Autodesk Fusion 360 part; units mm, degrees
note: some values were not read from the file. Chosen so that the rebuilt part matches the saved one: which pieces of a blend or face edit are solid.
(part 2 of 5)
  measures "d848" distance of L239.end L236.start
  measures "d854" distance of L244.start L244.end
  measures "d856" distance of L244.start L246.start
  measures "d862" distance of L237.end L256.start
  measures "d867" distance of L243.end L255.start
  measures "d868" distance of L255 L256
  measures "d884" distance of L393.end L393.start
  measures "d885" distance of L393.start L392.end
  measures "d887" distance of L392.start L392.end
  measures "d890" distance of L400.end L412.end
  measures "d896" distance of L150 L164
  measures "d921" distance of L177.start P8
  measures "d922" distance of L177 L458
  measures "d923" distance of L453 L458
  measures "d929" distance of L171.start L469.start
  measures "d930" distance of L171.start L23.end
  measures "d931" distance of P6 L472.start
  measures "d932" distance of P6 L473.end
  measures "d933" distance of L23 L24
  measures "d934" distance of L55.start L476.end
  measures "d937" distance of L7.start L57.end
  measures "d938" distance of L169 L479
  measures "d948" distance of L49.end L481.end
  measures "d949" distance of L482.start L482.end
  measures "d951" distance of L4.start L502.start
  measures "d956" distance of L172 L179
  measures "d1024" diameter of A16
  measures "d1025" diameter of A17
  measures "d1031" distance of L523 L524
sketch "Skizze2" plane through (0, 0, 0) normal (0, 0, 1) x (1, 0, 0)
  line L0 (0, 7.8901) -> (0, 0)
  line L1 (250, 0) -> (250, 8)
  line L2 (10, 8) -> (10, 0)
  line L3 (0, 0) -> (10, 0)
  line L4 (34.8226, 77.9951) -> (0.2007, 77.9951)
  line L5 (4.5, -4.5) -> (245.5, -4.5)
  line L6 (245.5, -245.5) -> (4.5, -245.5)
  line L7 (4.5, -245.5) -> (4.5, -4.5)
  circle A0 centre (7.5, -7.5) radius 1.5
  circle A1 centre (7.5, -7.5) radius 1.5
  circle A2 centre (7.7007, 70.4951) radius 1.5
  line L8 (240, 8) -> (10, 8)
  line L9 (240, 8) -> (240, 0)
  line L10 (0, 0) -> (0, 7.8901)
  line L11 (34.8226, 85.9951) -> (34.8226, 77.9951)
  line L12 (188.7268, 54.5014) -> (175.7207, 54.4951)
  line L13 (175.7207, 54.4951) -> (175.7307, 61.495)
  line L14 (175.7307, 61.495) -> (188.7307, 61.4887)
  line L15 (188.7307, 61.4887) -> (188.7268, 54.5014)
  line L16 (170.2913, 54.4924) -> (157.2903, 54.4861)
  line L17 (157.2903, 54.4861) -> (157.3035, 61.4861)
  line L18 (157.3035, 61.4861) -> (170.3035, 61.4612)
  line L19 (170.3035, 61.4612) -> (170.2913, 54.4924)
  line L20 (150.7313, 54.5045) -> (135.7242, 54.4951)
  line L21 (135.7242, 54.4951) -> (135.7359, 61.495)
  line L22 (135.7359, 61.495) -> (150.7359, 61.4856)
  line L23 (150.7359, 61.4856) -> (150.7313, 54.5045)
  line L24 (121.7084, 53.9672) -> (108.2084, 53.9709)
  line L25 (108.2084, 53.9709) -> (106.7182, 62.0188)
  line L26 (106.7182, 62.0188) -> (123.2182, 62.0233)
  line L27 (123.2182, 62.0233) -> (121.7084, 53.9672)
  line L28 (31.2246, 51.4951) -> (19.7246, 51.5056)
  line L29 (19.7246, 51.5056) -> (19.7282, 64.4845)
  line L30 (19.7282, 64.4845) -> (31.2439, 64.4951)
  line L31 (31.2439, 64.4951) -> (31.2246, 51.4951)
  circle A3 centre (18.2368, 25.8861) radius 4
  line L32 (211.2035, 57.9951) -> (16.1921, 57.9951)
  line L33 (95.7998, 57.9951) -> (36.1928, 58.2134)
  line L34 (36.1928, 58.2134) -> (36.1928, 40.7134)
  line L35 (36.1928, 40.7134) -> (95.799, 40.4951)
  line L36 (95.799, 40.4951) -> (95.7998, 57.9951)
  line L37 (47.3226, 85.9941) -> (47.3226, 77.9951)
  line L38 (90.3666, 86) -> (90.3677, 77.9951)
  line L39 (102.8855, 86) -> (102.8844, 77.9951)
  line L40 (145.9318, 86) -> (145.9321, 77.9951)
  line L41 (158.4356, 86) -> (158.4355, 77.9951)
  line L42 (201.4887, 86) -> (201.4887, 77.9951)
  line L43 (213.9898, 86) -> (213.9897, 77.9951)
  line L44 (47.3226, 85.9941) -> (34.8226, 85.9951)
  line L45 (102.8855, 86) -> (90.3666, 86)
  line L46 (158.4356, 86) -> (145.9318, 86)
  line L47 (213.9898, 86) -> (201.4887, 86)
  line L48 (-7.8996, 42.9426) -> (-7.8996, 7.8901)
  line L49 (-7.8996, 7.8901) -> (0, 7.8901)
  line L50 (250.1004, 77.9951) -> (258.1004, 77.9951)
  line L51 (258.1004, 8) -> (250, 8)
  circle A4 centre (242.7007, 70.4951) radius 1.5
  circle A5 centre (7.7007, 15.4951) radius 1.5
  circle A6 centre (242.7007, 15.4951) radius 1.5
  line L52 (213.9897, 77.9951) -> (250.1004, 77.9951)
  line L53 (213.9897, 77.9951) -> (250.1004, 77.9951)
  line L54 (158.4355, 77.9951) -> (201.4887, 77.9951)
  line L55 (158.4355, 77.9951) -> (201.4887, 77.9951)
  line L56 (102.8844, 77.9951) -> (145.9321, 77.9951)
  line L57 (47.3226, 77.9951) -> (90.3677, 77.9951)
  line L58 (102.8844, 77.9951) -> (145.9321, 77.9951)
  line L59 (0.2007, 77.9951) -> (34.8226, 77.9951)
  line L60 (47.3226, 77.9951) -> (90.3677, 77.9951)
  line L61 (0.1004, 369.8881) -> (-7.8996, 369.8881)
  line L62 (240.1004, 379.8881) -> (240.1004, 387.8881)
  line L63 (222.2222, 129.8881) -> (222.2222, 121.8881)
  line L64 (27.7778, 129.8881) -> (27.7778, 121.8881)
  line L65 (111.1111, 129.8881) -> (111.1111, 121.8881)
  line L66 (138.8889, 129.8881) -> (138.8889, 121.8881)
  line L67 (55.5556, 129.8881) -> (55.5556, 121.8881)
  line L68 (194.4444, 129.8881) -> (194.4444, 121.8881)
  circle A7 centre (7.6004, 137.3881) radius 1.5
  line L69 (166.6667, 129.8881) -> (166.6667, 121.8881)
  line L70 (0, 129.8881) -> (0, 121.8881)
  line L71 (83.3333, 129.8881) -> (83.3333, 121.8881)
  line L72 (-7.8996, 369.8881) -> (-7.8996, 139.8881)
  circle A8 centre (242.6004, 137.3881) radius 1.5
  line L73 (10.1004, 387.8881) -> (10.1004, 379.8881)
  circle A9 centre (242.6004, 372.3881) radius 1.5
  line L74 (240.1004, 387.8881) -> (10.1004, 387.8881)
  line L75 (0, 139.8881) -> (0, 129.8881)
  line L76 (-7.8996, 139.8881) -> (0, 139.8881)
  line L77 (240.1004, 379.8881) -> (250.1004, 379.8881)
  line L78 (0.1004, 379.8881) -> (10.1004, 379.8881)
  line L79 (0.1004, 379.8881) -> (0.1004, 369.8881)
  circle A10 centre (7.6004, 372.3881) radius 1.5
  line L80 (240, 0) -> (250, 0)
  line L81 (10, 0) -> (0, 0)
  circle A11 centre (7.5, -14.4118) radius 1.5
  circle A12 centre (7.5, -21.3235) radius 1.5
  circle A13 centre (7.5, -28.2353) radius 1.5
  circle A14 centre (7.5, -35.1471) radius 1.5
  circle A15 centre (7.5, -42.0588) radius 1.5
  circle A16 centre (7.5, -48.9706) radius 1.5
  circle A17 centre (7.5, -55.8824) radius 1.5
  circle A18 centre (7.5, -62.7941) radius 1.5
  circle A19 centre (7.5, -69.7059) radius 1.5
  circle A20 centre (7.5, -76.6176) radius 1.5
  circle A21 centre (7.5, -83.5294) radius 1.5
  circle A22 centre (7.5, -90.4412) radius 1.5
  circle A23 centre (7.5, -97.3529) radius 1.5
  circle A24 centre (7.5, -104.2647) radius 1.5
  circle A25 centre (7.5, -111.1765) radius 1.5
  circle A26 centre (7.5, -118.0882) radius 1.5
  circle A27 centre (7.5, -125) radius 1.5
  circle A28 centre (7.5, -131.9118) radius 1.5
  circle A29 centre (7.5, -138.8235) radius 1.5
  circle A30 centre (7.5, -145.7353) radius 1.5
  circle A31 centre (7.5, -152.6471) radius 1.5
  circle A32 centre (7.5, -159.5588) radius 1.5
  circle A33 centre (7.5, -166.4706) radius 1.5
  circle A34 centre (7.5, -173.3824) radius 1.5
  circle A35 centre (7.5, -180.2941) radius 1.5
  circle A36 centre (7.5, -187.2059) radius 1.5
  circle A37 centre (7.5, -194.1176) radius 1.5
  circle A38 centre (7.5, -201.0294) radius 1.5
  circle A39 centre (7.5, -207.9412) radius 1.5
  circle A40 centre (7.5, -214.8529) radius 1.5
  circle A41 centre (7.5, -221.7647) radius 1.5
  circle A42 centre (7.5, -228.6765) radius 1.5
  circle A43 centre (7.5, -235.5882) radius 1.5
  circle A44 centre (7.5, -242.5) radius 1.5
  circle A45 centre (170.8722, -303.1832) radius 1.75
  circle A46 centre (170.8722, -273.1832) radius 1.75
  circle A47 centre (95.8722, -273.1832) radius 1.75
  line L82 (245.5, -323.5) -> (4.5, -323.5)
  circle A48 centre (60.4769, -288.1832) radius 8
  line L83 (245.5, -262.5) -> (245.5, -323.5)
  circle A49 centre (79.6349, -288.1832) radius 3.25
  line L84 (97.6222, -276.9332) -> (169.1222, -276.9332)
  line L85 (169.1222, -299.4332) -> (97.6222, -299.4332)
  line L86 (169.1222, -276.9332) -> (169.1222, -299.4332)
  circle A50 centre (95.8722, -303.1832) radius 1.75
  line L87 (97.6222, -299.4332) -> (97.6222, -276.9332)
  line L88 (4.5, -323.5) -> (4.5, -262.5)
  line L89 (4.5, -262.5) -> (245.5, -262.5)
  circle A51 centre (7.5, -265.5) radius 1.5
  circle A52 centre (7.5, -265.5) radius 1.5
  circle A53 centre (19.25, -265.5) radius 1.5
  circle A54 centre (7.5, -274.6667) radius 1.5
  circle A55 centre (19.25, -274.6667) radius 1.5
  line L90 (-12.5, -4.5) -> (-73.5, -4.5)
  line L91 (-12.5, -245.5) -> (-12.5, -4.5)
  circle A56 centre (235, -284.5) radius 3
  circle A57 centre (235, -272.5) radius 3
  line L92 (229, -215.5) -> (231, -215.5)
  line L93 (231, -215.5) -> (231, -239.5)
  line L94 (231, -239.5) -> (229, -239.5)
  line L95 (229, -239.5) -> (229, -215.5)
  line L96 (240, -328) -> (10.0001, -328)
  circle A58 centre (31, -265.5) radius 1.5
  circle A59 centre (42.75, -265.5) radius 1.5
  circle A60 centre (54.5, -265.5) radius 1.5
  circle A61 centre (66.25, -265.5) radius 1.5
  circle A62 centre (78, -265.5) radius 1.5
  circle A63 centre (89.75, -265.5) radius 1.5
  circle A64 centre (101.5, -265.5) radius 1.5
  circle A65 centre (125, -265.5) radius 1.5
  circle A66 centre (136.75, -265.5) radius 1.5
  circle A67 centre (148.5, -265.5) radius 1.5
  circle A68 centre (183.75, -265.5) radius 1.5
  circle A69 centre (195.5, -265.5) radius 1.5
  circle A70 centre (207.25, -265.5) radius 1.5
  circle A71 centre (31, -274.6667) radius 1.5
  circle A72 centre (42.75, -274.6667) radius 1.5
  circle A73 centre (183.75, -274.6667) radius 1.5
  circle A74 centre (195.5, -274.6667) radius 1.5
  circle A75 centre (207.25, -274.6667) radius 1.5
  circle A76 centre (7.5, -283.8333) radius 1.5
  circle A77 centre (19.25, -283.8333) radius 1.5
  circle A78 centre (31, -283.8333) radius 1.5
  circle A79 centre (195.5, -283.8333) radius 1.5
  circle A80 centre (207.25, -283.8333) radius 1.5
  circle A81 centre (7.5, -293) radius 1.5
  circle A82 centre (19.25, -293) radius 1.5
  circle A83 centre (31, -293) radius 1.5
  circle A84 centre (195.5, -293) radius 1.5
  circle A85 centre (207.25, -293) radius 1.5
  circle A86 centre (7.5, -302.1667) radius 1.5
  circle A87 centre (19.25, -302.1667) radius 1.5
  circle A88 centre (31, -302.1667) radius 1.5
  circle A89 centre (42.75, -302.1667) radius 1.5
  circle A90 centre (183.75, -302.1667) radius 1.5
  circle A91 centre (195.5, -302.1667) radius 1.5
  circle A92 centre (207.25, -302.1667) radius 1.5
  circle A93 centre (7.5, -311.3333) radius 1.5
  circle A94 centre (19.25, -311.3333) radius 1.5
  circle A95 centre (31, -311.3333) radius 1.5
  circle A96 centre (42.75, -311.3333) radius 1.5
  circle A97 centre (54.5, -311.3333) radius 1.5
  circle A98 centre (66.25, -311.3333) radius 1.5
  circle A99 centre (78, -311.3333) radius 1.5
  circle A100 centre (89.75, -311.3333) radius 1.5
  circle A101 centre (101.5, -311.3333) radius 1.5
  circle A102 centre (113.25, -311.3333) radius 1.5
  circle A103 centre (125, -311.3333) radius 1.5
  circle A104 centre (136.75, -311.3333) radius 1.5
  circle A105 centre (148.5, -311.3333) radius 1.5
  circle A106 centre (160.25, -311.3333) radius 1.5
  circle A107 centre (172, -311.3333) radius 1.5
  circle A108 centre (183.75, -311.3333) radius 1.5
  circle A109 centre (195.5, -311.3333) radius 1.5
  circle A110 centre (207.25, -311.3333) radius 1.5
  circle A111 centre (7.5, -320.5) radius 1.5
  circle A112 centre (19.25, -320.5) radius 1.5
  circle A113 centre (31, -320.5) radius 1.5
  circle A114 centre (42.75, -320.5) radius 1.5
  circle A115 centre (54.5, -320.5) radius 1.5
  circle A116 centre (66.25, -320.5) radius 1.5
  circle A117 centre (78, -320.5) radius 1.5
  circle A118 centre (89.75, -320.5) radius 1.5
  circle A119 centre (101.5, -320.5) radius 1.5
  circle A120 centre (113.25, -320.5) radius 1.5
  circle A121 centre (125, -320.5) radius 1.5
  circle A122 centre (136.75, -320.5) radius 1.5
  circle A123 centre (148.5, -320.5) radius 1.5
  circle A124 centre (160.25, -320.5) radius 1.5
  circle A125 centre (172, -320.5) radius 1.5
  circle A126 centre (183.75, -320.5) radius 1.5
  circle A127 centre (195.5, -320.5) radius 1.5
  circle A128 centre (207.25, -320.5) radius 1.5
  line L97 (0, -250) -> (27.7778, -250)
  circle A129 centre (242.5, -265.5) radius 1.5
  circle A130 centre (219, -274.6667) radius 1.5
  circle A131 centre (242.5, -274.6667) radius 1.5
  circle A132 centre (219, -283.8333) radius 1.5
  circle A133 centre (242.5, -283.8333) radius 1.5
  circle A134 centre (219, -293) radius 1.5
  circle A135 centre (230.75, -293) radius 1.5
  circle A136 centre (242.5, -293) radius 1.5
  circle A137 centre (219, -302.1667) radius 1.5
  circle A138 centre (230.75, -302.1667) radius 1.5
  circle A139 centre (242.5, -302.1667) radius 1.5
  circle A140 centre (219, -311.3333) radius 1.5
  circle A141 centre (230.75, -311.3333) radius 1.5
  circle A142 centre (242.5, -311.3333) radius 1.5
  circle A143 centre (219, -320.5) radius 1.5
  circle A144 centre (230.75, -320.5) radius 1.5
  circle A145 centre (242.5, -320.5) radius 1.5
  circle A146 centre (219, -265.5) radius 1.5
  circle A147 centre (230.75, -265.5) radius 1.5
  circle A148 centre (-15.5, -7.5) radius 1.5
  circle A149 centre (-15.5, -7.5) radius 1.5
  circle A150 centre (-70.5, -7.5) radius 1.5
  circle A151 centre (-15.5, -242.5) radius 1.5
  circle A152 centre (-70.5, -242.5) radius 1.5
  line L98 (-71, -250) -> (-64, -250)
  line L99 (-8, -27.7778) -> (-8, -55.5556)
  line L100 (-27.4566, -13.5) -> (-41.8362, -13.5)
  line L101 (-56.2158, -13.5) -> (-64.5, -13.5)
  line L102 (-21.5, -31.178) -> (-21.5, -18.678)
  line L103 (-64.5, -13.5) -> (-64.5, -18.7987)
  line L104 (-21.5, -56.178) -> (-21.5, -43.678)
  line L105 (-64.5, -31.2987) -> (-64.5, -43.7987)
  line L106 (-21.5, -81.178) -> (-21.5, -68.678)
  line L107 (-64.5, -56.2987) -> (-64.5, -68.7987)
  line L108 (-21.5, -106.178) -> (-21.5, -93.678)
  line L109 (-64.5, -93.7987) -> (-21.5, -131.178)
  line L110 (-64.5, -156.2987) -> (-21.5, -193.678)
  line L111 (-64.5, -218.7987) -> (-51.0392, -230.5)
  line L112 (-64.5, -206.2987) -> (-36.6596, -230.5)
  line L113 (-64.5, -193.7987) -> (-22.28, -230.5)
  line L114 (-64.5, -181.2987) -> (-21.5, -218.678)
  line L115 (-64.5, -168.7987) -> (-21.5, -206.178)
  line L116 (-64.5, -143.7987) -> (-21.5, -181.178)
  line L117 (-64.5, -131.2987) -> (-21.5, -168.678)
  line L118 (-64.5, -118.7987) -> (-21.5, -156.178)
  line L119 (-64.5, -106.2987) -> (-21.5, -143.678)
  line L120 (-64.5, -81.2987) -> (-21.5, -118.678)
  line L121 (-64.5, -68.7987) -> (-21.5, -106.178)
  line L122 (-64.5, -56.2987) -> (-21.5, -93.678)
  line L123 (-64.5, -43.7987) -> (-21.5, -81.178)
  line L124 (-64.5, -31.2987) -> (-21.5, -68.678)
  line L125 (-64.5, -18.7987) -> (-21.5, -56.178)
  line L126 (-21.5, -131.178) -> (-21.5, -118.678)
  line L127 (-21.5, -156.178) -> (-21.5, -143.678)
  line L128 (-21.5, -181.178) -> (-21.5, -168.678)
  line L129 (-21.5, -230.5) -> (-21.5, -218.678)
  line L130 (-21.5, -206.178) -> (-21.5, -193.678)
  line L131 (-51.0392, -230.5) -> (-36.6596, -230.5)
  line L132 (-22.28, -230.5) -> (-21.5, -230.5)
  line L133 (-64.5, -206.2987) -> (-64.5, -218.7987)
  line L134 (-64.5, -181.2987) -> (-64.5, -193.7987)
  line L135 (-64.5, -156.2987) -> (-64.5, -168.7987)
  line L136 (-64.5, -131.2987) -> (-64.5, -143.7987)
  line L137 (-64.5, -81.2987) -> (-64.5, -93.7987)
  line L138 (-64.5, -106.2987) -> (-64.5, -118.7987)
  line L139 (-41.8362, -13.5) -> (-21.5, -31.178)
  line L140 (-56.2158, -13.5) -> (-21.5, -43.678)
  line L141 (-27.4566, -13.5) -> (-21.5, -18.678)
  circle A153 centre (265.5, -242.5) radius 1.5
  circle A154 centre (265.5, -242.5) radius 1.5
  circle A155 centre (276.5, -242.5) radius 1.5
  circle A156 centre (276.5, -242.5) radius 1.5
  circle A157 centre (265.5, -229.4444) radius 1.5
  circle A158 centre (265.5, -229.4444) radius 1.5
  circle A159 centre (276.5, -229.4444) radius 1.5
  circle A160 centre (276.5, -229.4444) radius 1.5
  line L142 (262.5, -245.5) -> (323.5, -245.5)
  line L143 (323.5, -245.5) -> (323.5, -4.5)
  line L144 (323.5, -4.5) -> (262.5, -4.5)
  line L145 (262.5, -4.5) -> (262.5, -245.5)
  line L146 (271.7317, -182.5048) -> (315.1722, -182.5048)
  line L147 (315.1722, -182.5048) -> (315.1722, -170.5048)
  line L148 (315.1722, -170.5048) -> (271.7317, -170.5048)
  line L149 (271.7317, -170.5048) -> (271.7317, -182.5048)
  circle A161 centre (287.5, -242.5) radius 1.5
  circle A162 centre (287.5, -242.5) radius 1.5
  circle A163 centre (298.5, -242.5) radius 1.5
  circle A164 centre (298.5, -242.5) radius 1.5
  circle A165 centre (309.5, -242.5) radius 1.5
  circle A166 centre (309.5, -242.5) radius 1.5
  circle A167 centre (287.5, -229.4444) radius 1.5
  circle A168 centre (287.5, -229.4444) radius 1.5
  circle A169 centre (298.5, -229.4444) radius 1.5
  circle A170 centre (298.5, -229.4444) radius 1.5
  circle A171 centre (309.5, -229.4444) radius 1.5
  circle A172 centre (309.5, -229.4444) radius 1.5
  circle A173 centre (265.5, -216.3889) radius 1.5
  circle A174 centre (265.5, -216.3889) radius 1.5
  circle A175 centre (276.5, -216.3889) radius 1.5
  circle A176 centre (276.5, -216.3889) radius 1.5
  circle A177 centre (287.5, -216.3889) radius 1.5
  circle A178 centre (287.5, -216.3889) radius 1.5
  circle A179 centre (298.5, -216.3889) radius 1.5
  circle A180 centre (298.5, -216.3889) radius 1.5
  circle A181 centre (309.5, -216.3889) radius 1.5
  circle A182 centre (309.5, -216.3889) radius 1.5
  circle A183 centre (265.5, -203.3333) radius 1.5
  circle A184 centre (265.5, -203.3333) radius 1.5
  circle A185 centre (276.5, -203.3333) radius 1.5
  circle A186 centre (276.5, -203.3333) radius 1.5
  circle A187 centre (287.5, -203.3333) radius 1.5
  circle A188 centre (287.5, -203.3333) radius 1.5
  circle A189 centre (298.5, -203.3333) radius 1.5
  circle A190 centre (298.5, -203.3333) radius 1.5
  circle A191 centre (309.5, -203.3333) radius 1.5
  circle A192 centre (309.5, -203.3333) radius 1.5
  circle A193 centre (265.5, -190.2778) radius 1.5
  circle A194 centre (265.5, -190.2778) radius 1.5
  circle A195 centre (276.5, -190.2778) radius 1.5
  circle A196 centre (276.5, -190.2778) radius 1.5
  circle A197 centre (287.5, -190.2778) radius 1.5
  circle A198 centre (287.5, -190.2778) radius 1.5
  circle A199 centre (298.5, -190.2778) radius 1.5
  circle A200 centre (298.5, -190.2778) radius 1.5
  circle A201 centre (309.5, -190.2778) radius 1.5
  circle A202 centre (309.5, -190.2778) radius 1.5
  circle A203 centre (265.5, -177.2222) radius 1.5
  circle A204 centre (265.5, -177.2222) radius 1.5
  circle A205 centre (265.5, -164.1667) radius 1.5
  circle A206 centre (265.5, -164.1667) radius 1.5
  circle A207 centre (276.5, -164.1667) radius 1.5
  circle A208 centre (276.5, -164.1667) radius 1.5
  circle A209 centre (287.5, -164.1667) radius 1.5
  circle A210 centre (287.5, -164.1667) radius 1.5
  circle A211 centre (298.5, -164.1667) radius 1.5
  circle A212 centre (298.5, -164.1667) radius 1.5
  circle A213 centre (309.5, -164.1667) radius 1.5
  circle A214 centre (309.5, -164.1667) radius 1.5
  circle A215 centre (265.5, -151.1111) radius 1.5
  circle A216 centre (265.5, -151.1111) radius 1.5
  circle A217 centre (276.5, -151.1111) radius 1.5
  circle A218 centre (276.5, -151.1111) radius 1.5
  circle A219 centre (287.5, -151.1111) radius 1.5
  circle A220 centre (287.5, -151.1111) radius 1.5
  circle A221 centre (298.5, -151.1111) radius 1.5
  circle A222 centre (298.5, -151.1111) radius 1.5
  circle A223 centre (309.5, -151.1111) radius 1.5
  circle A224 centre (309.5, -151.1111) radius 1.5
  circle A225 centre (265.5, -138.0556) radius 1.5
  circle A226 centre (265.5, -138.0556) radius 1.5
  circle A227 centre (276.5, -138.0556) radius 1.5
  circle A228 centre (276.5, -138.0556) radius 1.5
  circle A229 centre (287.5, -138.0556) radius 1.5
  circle A230 centre (287.5, -138.0556) radius 1.5
  circle A231 centre (298.5, -138.0556) radius 1.5
  circle A232 centre (298.5, -138.0556) radius 1.5
  circle A233 centre (309.5, -138.0556) radius 1.5
  circle A234 centre (309.5, -138.0556) radius 1.5
  circle A235 centre (265.5, -125) radius 1.5
  circle A236 centre (265.5, -125) radius 1.5
  circle A237 centre (276.5, -125) radius 1.5
  circle A238 centre (276.5, -125) radius 1.5
  circle A239 centre (287.5, -125) radius 1.5
  circle A240 centre (287.5, -125) radius 1.5
  circle A241 centre (298.5, -125) radius 1.5
  circle A242 centre (298.5, -125) radius 1.5
  circle A243 centre (309.5, -125) radius 1.5
  circle A244 centre (309.5, -125) radius 1.5
  circle A245 centre (265.5, -111.9444) radius 1.5
  circle A246 centre (265.5, -111.9444) radius 1.5
  circle A247 centre (276.5, -111.9444) radius 1.5
  circle A248 centre (276.5, -111.9444) radius 1.5
  circle A249 centre (287.5, -111.9444) radius 1.5
  circle A250 centre (287.5, -111.9444) radius 1.5
  circle A251 centre (298.5, -111.9444) radius 1.5
  circle A252 centre (298.5, -111.9444) radius 1.5
  circle A253 centre (309.5, -111.9444) radius 1.5
  circle A254 centre (309.5, -111.9444) radius 1.5
  circle A255 centre (265.5, -98.8889) radius 1.5
  circle A256 centre (265.5, -98.8889) radius 1.5
  circle A257 centre (276.5, -98.8889) radius 1.5
  circle A258 centre (276.5, -98.8889) radius 1.5
  circle A259 centre (287.5, -98.8889) radius 1.5
  circle A260 centre (287.5, -98.8889) radius 1.5
  circle A261 centre (298.5, -98.8889) radius 1.5
  circle A262 centre (298.5, -98.8889) radius 1.5
  circle A263 centre (309.5, -98.8889) radius 1.5
  circle A264 centre (309.5, -98.8889) radius 1.5
  circle A265 centre (265.5, -85.8333) radius 1.5
  circle A266 centre (265.5, -85.8333) radius 1.5
  circle A267 centre (276.5, -85.8333) radius 1.5
  circle A268 centre (276.5, -85.8333) radius 1.5
  circle A269 centre (287.5, -85.8333) radius 1.5
  circle A270 centre (287.5, -85.8333) radius 1.5
  circle A271 centre (298.5, -85.8333) radius 1.5
  circle A272 centre (298.5, -85.8333) radius 1.5
  circle A273 centre (309.5, -85.8333) radius 1.5
  circle A274 centre (309.5, -85.8333) radius 1.5
  circle A275 centre (265.5, -72.7778) radius 1.5
  circle A276 centre (265.5, -72.7778) radius 1.5
  circle A277 centre (276.5, -72.7778) radius 1.5
  circle A278 centre (276.5, -72.7778) radius 1.5
  circle A279 centre (287.5, -72.7778) radius 1.5
  circle A280 centre (287.5, -72.7778) radius 1.5
  circle A281 centre (298.5, -72.7778) radius 1.5
  circle A282 centre (298.5, -72.7778) radius 1.5
  circle A283 centre (309.5, -72.7778) radius 1.5
  circle A284 centre (309.5, -72.7778) radius 1.5
  circle A285 centre (265.5, -59.7222) radius 1.5
  circle A286 centre (265.5, -59.7222) radius 1.5
  circle A287 centre (276.5, -59.7222) radius 1.5
  circle A288 centre (276.5, -59.7222) radius 1.5
  circle A289 centre (287.5, -59.7222) radius 1.5
  circle A290 centre (287.5, -59.7222) radius 1.5
  circle A291 centre (298.5, -59.7222) radius 1.5
  circle A292 centre (298.5, -59.7222) radius 1.5
  circle A293 centre (309.5, -59.7222) radius 1.5
  circle A294 centre (309.5, -59.7222) radius 1.5
  circle A295 centre (265.5, -46.6667) radius 1.5
  circle A296 centre (265.5, -46.6667) radius 1.5
  circle A297 centre (276.5, -46.6667) radius 1.5
  circle A298 centre (276.5, -46.6667) radius 1.5
  circle A299 centre (287.5, -46.6667) radius 1.5
  circle A300 centre (287.5, -46.6667) radius 1.5
  circle A301 centre (298.5, -46.6667) radius 1.5
  circle A302 centre (298.5, -46.6667) radius 1.5
  circle A303 centre (309.5, -46.6667) radius 1.5
  circle A304 centre (309.5, -46.6667) radius 1.5
  circle A305 centre (265.5, -33.6111) radius 1.5
  circle A306 centre (265.5, -33.6111) radius 1.5
  circle A307 centre (276.5, -33.6111) radius 1.5
  circle A308 centre (276.5, -33.6111) radius 1.5
  circle A309 centre (287.5, -33.6111) radius 1.5
  circle A310 centre (287.5, -33.6111) radius 1.5
  circle A311 centre (298.5, -33.6111) radius 1.5
  circle A312 centre (298.5, -33.6111) radius 1.5
  circle A313 centre (309.5, -33.6111) radius 1.5
  circle A314 centre (309.5, -33.6111) radius 1.5
  circle A315 centre (320.5, -242.5) radius 1.5
  circle A316 centre (320.5, -242.5) radius 1.5
  circle A317 centre (320.5, -229.4444) radius 1.5
  circle A318 centre (320.5, -229.4444) radius 1.5
  circle A319 centre (320.5, -216.3889) radius 1.5
  circle A320 centre (320.5, -216.3889) radius 1.5
  circle A321 centre (320.5, -203.3333) radius 1.5
  circle A322 centre (320.5, -203.3333) radius 1.5
  circle A323 centre (320.5, -190.2778) radius 1.5
  circle A324 centre (320.5, -190.2778) radius 1.5
  circle A325 centre (320.5, -177.2222) radius 1.5
  circle A326 centre (320.5, -177.2222) radius 1.5
  circle A327 centre (320.5, -164.1667) radius 1.5
  circle A328 centre (320.5, -164.1667) radius 1.5
  circle A329 centre (320.5, -151.1111) radius 1.5
  circle A330 centre (320.5, -151.1111) radius 1.5
  circle A331 centre (320.5, -138.0556) radius 1.5
  circle A332 centre (320.5, -138.0556) radius 1.5
  circle A333 centre (320.5, -125) radius 1.5
  circle A334 centre (320.5, -125) radius 1.5
  circle A335 centre (320.5, -111.9444) radius 1.5
  circle A336 centre (320.5, -111.9444) radius 1.5
  circle A337 centre (320.5, -98.8889) radius 1.5
  circle A338 centre (320.5, -98.8889) radius 1.5
  circle A339 centre (320.5, -85.8333) radius 1.5
  circle A340 centre (320.5, -85.8333) radius 1.5
  circle A341 centre (320.5, -72.7778) radius 1.5
  circle A342 centre (320.5, -72.7778) radius 1.5
  circle A343 centre (320.5, -59.7222) radius 1.5
  circle A344 centre (320.5, -59.7222) radius 1.5
  circle A345 centre (320.5, -46.6667) radius 1.5
  circle A346 centre (320.5, -46.6667) radius 1.5
  circle A347 centre (320.5, -33.6111) radius 1.5
  circle A348 centre (320.5, -33.6111) radius 1.5
  circle A349 centre (265.5, -20.5556) radius 1.5
  circle A350 centre (265.5, -20.5556) radius 1.5
  circle A351 centre (276.5, -20.5556) radius 1.5
  circle A352 centre (276.5, -20.5556) radius 1.5
  circle A353 centre (287.5, -20.5556) radius 1.5
  circle A354 centre (287.5, -20.5556) radius 1.5
  circle A355 centre (298.5, -20.5556) radius 1.5
  circle A356 centre (298.5, -20.5556) radius 1.5
  circle A357 centre (309.5, -20.5556) radius 1.5
  circle A358 centre (309.5, -20.5556) radius 1.5
  circle A359 centre (320.5, -20.5556) radius 1.5
  circle A360 centre (320.5, -20.5556) radius 1.5
  circle A361 centre (265.5, -7.5) radius 1.5
  circle A362 centre (265.5, -7.5) radius 1.5
  circle A363 centre (276.5, -7.5) radius 1.5
  circle A364 centre (276.5, -7.5) radius 1.5
  circle A365 centre (287.5, -7.5) radius 1.5
  circle A366 centre (287.5, -7.5) radius 1.5
  circle A367 centre (298.5, -7.5) radius 1.5
  circle A368 centre (298.5, -7.5) radius 1.5
  circle A369 centre (309.5, -7.5) radius 1.5
  circle A370 centre (309.5, -7.5) radius 1.5
  circle A371 centre (320.5, -7.5) radius 1.5
  circle A372 centre (320.5, -7.5) radius 1.5
  line L150 (0, 0) -> (0, -27.7778)
  line L151 (27.7778, 121.8881) -> (55.5556, 121.8881)
  line L152 (83.3333, 121.8881) -> (111.1111, 121.8881)
  line L153 (138.8889, 121.8881) -> (166.6667, 121.8881)
  line L154 (194.4444, 121.8881) -> (222.2222, 121.8881)
  line L155 (222.2222, 129.8881) -> (250.1004, 129.8881)
  line L156 (166.6667, 129.8881) -> (194.4444, 129.8881)
  line L157 (111.1111, 129.8881) -> (138.8889, 129.8881)
  line L158 (0, 129.8881) -> (27.7778, 129.8881)
  line L159 (55.5556, 129.8881) -> (83.3333, 129.8881)
  line L160 (429.9679, -3) -> (673.9679, -3)
  line L161 (673.9679, -3) -> (673.9679, -247)
  line L162 (673.9679, -247) -> (429.9679, -247)
  line L163 (429.9679, -247) -> (429.9679, -3)
  line L164 (432.9679, -6) -> (670.9679, -6)
  line L165 (670.9679, -6) -> (670.9679, -244)
  line L166 (670.9679, -244) -> (432.9679, -244)
  line L167 (432.9679, -244) -> (432.9679, -6)
  line L168 (426.9679, -83.3333) -> (426.9679, -55.5556)
  line L169 (649.1901, 0) -> (676.9679, 0)
  line L170 (-73.5, -4.5) -> (-73.5, -245.5)
  line L171 (-73.5, -245.5) -> (-12.5, -245.5)
  line L172 (-15, -250) -> (-8, -250)
  line L173 (34.8226, 126.8881) -> (47.3226, 126.8881)
  line L174 (47.3226, 126.8881) -> (47.3226, 123.8881)
  line L175 (47.3226, 123.8881) -> (34.8226, 123.8881)
  line L176 (34.8226, 123.8881) -> (34.8226, 126.8881)
  line L177 (102.8908, 123.8881) -> (90.3614, 123.8881)
  line L178 (102.8912, 126.8881) -> (102.8908, 123.8881)
  line L179 (90.3614, 123.8881) -> (90.361, 126.8881)
  line L180 (90.361, 126.8881) -> (102.8912, 126.8881)
  line L181 (158.4361, 123.8881) -> (145.9305, 123.8881)
  line L182 (158.4362, 126.8881) -> (158.4361, 123.8881)
  line L183 (145.9305, 123.8881) -> (145.9304, 126.8881)
  line L184 (145.9304, 126.8881) -> (158.4362, 126.8881)
  line L185 (213.9901, 123.8881) -> (201.4885, 123.8881)
  line L186 (213.9901, 126.8881) -> (213.9901, 123.8881)
  line L187 (201.4885, 123.8881) -> (201.4885, 126.8881)
  line L188 (201.4885, 126.8881) -> (213.9901, 126.8881)
  line L189 (250.1004, 70.2173) -> (258.1004, 70.2173)
  line L190 (250.1004, 62.4395) -> (258.1004, 62.4395)
  line L191 (250.1004, 54.6617) -> (258.1004, 54.6617)
  line L192 (250.1004, 46.8839) -> (258.1004, 46.8839)
  line L193 (250.1004, 39.1062) -> (258.1004, 39.1062)
  line L194 (250.1004, 31.3284) -> (258.1004, 31.3284)
  line L195 (250.1004, 23.5506) -> (258.1004, 23.5506)
  line L196 (250.1004, 15.7728) -> (258.1004, 15.7728)
  line L197 (250.1004, 7.9951) -> (258.1004, 7.9951)
  line L198 (258.1004, 15.7728) -> (258.1004, 8)
  line L199 (258.1004, 77.9951) -> (258.1004, 70.2173)
  line L200 (258.1004, 62.4395) -> (258.1004, 54.6617)
  line L201 (258.1004, 46.8839) -> (258.1004, 39.1062)
  line L202 (258.1004, 31.3284) -> (258.1004, 23.5506)
  line L203 (250.1004, 70.2173) -> (250.1004, 62.4395)
  line L204 (250.1004, 54.6617) -> (250.1004, 46.8839)
  line L205 (250.1004, 39.1062) -> (250.1004, 31.3284)
  line L206 (250.1004, 23.5506) -> (250.1004, 15.7728)
  line L207 (250, 0) -> (258, 0)
  line L208 (426.9679, -27.7778) -> (426.9679, 0)
  line L209 (426.9679, 0) -> (454.7457, 0)
  circle A373 centre (14.4118, -7.5) radius 1.5
  circle A374 centre (21.3235, -7.5) radius 1.5
  circle A375 centre (28.2353, -7.5) radius 1.5
  circle A376 centre (35.1471, -7.5) radius 1.5
  circle A377 centre (42.0588, -7.5) radius 1.5
  circle A378 centre (48.9706, -7.5) radius 1.5
  circle A379 centre (55.8824, -7.5) radius 1.5
  circle A380 centre (62.7941, -7.5) radius 1.5
  circle A381 centre (69.7059, -7.5) radius 1.5
  circle A382 centre (76.6176, -7.5) radius 1.5
  circle A383 centre (83.5294, -7.5) radius 1.5
  circle A384 centre (90.4412, -7.5) radius 1.5
  circle A385 centre (97.3529, -7.5) radius 1.5
  circle A386 centre (104.2647, -7.5) radius 1.5
  circle A387 centre (111.1765, -7.5) radius 1.5
  circle A388 centre (118.0882, -7.5) radius 1.5
  circle A389 centre (125, -7.5) radius 1.5
  circle A390 centre (131.9118, -7.5) radius 1.5
  circle A391 centre (138.8235, -7.5) radius 1.5
  circle A392 centre (145.7353, -7.5) radius 1.5
  circle A393 centre (152.6471, -7.5) radius 1.5
  circle A394 centre (159.5588, -7.5) radius 1.5
  circle A395 centre (166.4706, -7.5) radius 1.5
  circle A396 centre (173.3824, -7.5) radius 1.5
  circle A397 centre (180.2941, -7.5) radius 1.5
  circle A398 centre (187.2059, -7.5) radius 1.5
  circle A399 centre (194.1176, -7.5) radius 1.5
  circle A400 centre (201.0294, -7.5) radius 1.5
  circle A401 centre (207.9412, -7.5) radius 1.5
  circle A402 centre (214.8529, -7.5) radius 1.5
  circle A403 centre (221.7647, -7.5) radius 1.5
  circle A404 centre (228.6765, -7.5) radius 1.5
  circle A405 centre (235.5882, -7.5) radius 1.5
  circle A406 centre (242.5, -7.5) radius 1.5
  circle A407 centre (14.4118, -14.4118) radius 1.5
  circle A408 centre (21.3235, -14.4118) radius 1.5
  circle A409 centre (28.2353, -14.4118) radius 1.5
  circle A410 centre (35.1471, -14.4118) radius 1.5
  circle A411 centre (42.0588, -14.4118) radius 1.5
  circle A412 centre (48.9706, -14.4118) radius 1.5
  circle A413 centre (55.8824, -14.4118) radius 1.5
  circle A414 centre (62.7941, -14.4118) radius 1.5
  circle A415 centre (69.7059, -14.4118) radius 1.5
  circle A416 centre (76.6176, -14.4118) radius 1.5
  circle A417 centre (83.5294, -14.4118) radius 1.5
  circle A418 centre (90.4412, -14.4118) radius 1.5
  circle A419 centre (97.3529, -14.4118) radius 1.5
  circle A420 centre (104.2647, -14.4118) radius 1.5
  circle A421 centre (111.1765, -14.4118) radius 1.5
  circle A422 centre (118.0882, -14.4118) radius 1.5
  circle A423 centre (125, -14.4118) radius 1.5
  circle A424 centre (131.9118, -14.4118) radius 1.5
  circle A425 centre (138.8235, -14.4118) radius 1.5
  circle A426 centre (145.7353, -14.4118) radius 1.5
  circle A427 centre (152.6471, -14.4118) radius 1.5
  circle A428 centre (159.5588, -14.4118) radius 1.5
  circle A429 centre (166.4706, -14.4118) radius 1.5
  circle A430 centre (173.3824, -14.4118) radius 1.5
  circle A431 centre (180.2941, -14.4118) radius 1.5
  circle A432 centre (187.2059, -14.4118) radius 1.5
  circle A433 centre (194.1176, -14.4118) radius 1.5
  circle A434 centre (201.0294, -14.4118) radius 1.5
  circle A435 centre (207.9412, -14.4118) radius 1.5
  circle A436 centre (214.8529, -14.4118) radius 1.5
  circle A437 centre (221.7647, -14.4118) radius 1.5
  circle A438 centre (228.6765, -14.4118) radius 1.5
  circle A439 centre (235.5882, -14.4118) radius 1.5
  circle A440 centre (242.5, -14.4118) radius 1.5
  circle A441 centre (14.4118, -21.3235) radius 1.5
  circle A442 centre (21.3235, -21.3235) radius 1.5
  circle A443 centre (28.2353, -21.3235) radius 1.5
  circle A444 centre (35.1471, -21.3235) radius 1.5
  circle A445 centre (42.0588, -21.3235) radius 1.5
  circle A446 centre (48.9706, -21.3235) radius 1.5
  circle A447 centre (55.8824, -21.3235) radius 1.5
  circle A448 centre (62.7941, -21.3235) radius 1.5
  circle A449 centre (69.7059, -21.3235) radius 1.5
  circle A450 centre (76.6176, -21.3235) radius 1.5
  circle A451 centre (83.5294, -21.3235) radius 1.5
  circle A452 centre (90.4412, -21.3235) radius 1.5
  circle A453 centre (97.3529, -21.3235) radius 1.5
  circle A454 centre (104.2647, -21.3235) radius 1.5
  circle A455 centre (111.1765, -21.3235) radius 1.5
  circle A456 centre (118.0882, -21.3235) radius 1.5
  circle A457 centre (125, -21.3235) radius 1.5
  circle A458 centre (131.9118, -21.3235) radius 1.5
  circle A459 centre (138.8235, -21.3235) radius 1.5
  circle A460 centre (145.7353, -21.3235) radius 1.5
  circle A461 centre (152.6471, -21.3235) radius 1.5
  circle A462 centre (159.5588, -21.3235) radius 1.5
  circle A463 centre (166.4706, -21.3235) radius 1.5
  circle A464 centre (173.3824, -21.3235) radius 1.5
  circle A465 centre (180.2941, -21.3235) radius 1.5
  circle A466 centre (187.2059, -21.3235) radius 1.5
  circle A467 centre (194.1176, -21.3235) radius 1.5
  circle A468 centre (201.0294, -21.3235) radius 1.5
  circle A469 centre (207.9412, -21.3235) radius 1.5
  circle A470 centre (214.8529, -21.3235) radius 1.5
  circle A471 centre (221.7647, -21.3235) radius 1.5
  circle A472 centre (228.6765, -21.3235) radius 1.5
  circle A473 centre (235.5882, -21.3235) radius 1.5
  circle A474 centre (242.5, -21.3235) radius 1.5
  circle A475 centre (14.4118, -28.2353) radius 1.5
  circle A476 centre (21.3235, -28.2353) radius 1.5
  circle A477 centre (28.2353, -28.2353) radius 1.5
  circle A478 centre (35.1471, -28.2353) radius 1.5
  circle A479 centre (42.0588, -28.2353) radius 1.5
  circle A480 centre (48.9706, -28.2353) radius 1.5
  circle A481 centre (55.8824, -28.2353) radius 1.5
  circle A482 centre (62.7941, -28.2353) radius 1.5
  circle A483 centre (69.7059, -28.2353) radius 1.5
  circle A484 centre (76.6176, -28.2353) radius 1.5
  circle A485 centre (83.5294, -28.2353) radius 1.5
  circle A486 centre (90.4412, -28.2353) radius 1.5
  circle A487 centre (97.3529, -28.2353) radius 1.5
  circle A488 centre (104.2647, -28.2353) radius 1.5
  circle A489 centre (111.1765, -28.2353) radius 1.5
  circle A490 centre (118.0882, -28.2353) radius 1.5
  circle A491 centre (125, -28.2353) radius 1.5
  circle A492 centre (131.9118, -28.2353) radius 1.5
  circle A493 centre (138.8235, -28.2353) radius 1.5
  circle A494 centre (145.7353, -28.2353) radius 1.5
  circle A495 centre (152.6471, -28.2353) radius 1.5
  circle A496 centre (159.5588, -28.2353) radius 1.5
  circle A497 centre (166.4706, -28.2353) radius 1.5
  circle A498 centre (173.3824, -28.2353) radius 1.5
  circle A499 centre (180.2941, -28.2353) radius 1.5
  circle A500 centre (187.2059, -28.2353) radius 1.5
  circle A501 centre (194.1176, -28.2353) radius 1.5
  circle A502 centre (201.0294, -28.2353) radius 1.5
  circle A503 centre (207.9412, -28.2353) radius 1.5
  circle A504 centre (214.8529, -28.2353) radius 1.5
  circle A505 centre (221.7647, -28.2353) radius 1.5
  circle A506 centre (228.6765, -28.2353) radius 1.5
  circle A507 centre (235.5882, -28.2353) radius 1.5
  circle A508 centre (242.5, -28.2353) radius 1.5
  circle A509 centre (14.4118, -35.1471) radius 1.5
  circle A510 centre (21.3235, -35.1471) radius 1.5
  circle A511 centre (28.2353, -35.1471) radius 1.5
  circle A512 centre (35.1471, -35.1471) radius 1.5
  circle A513 centre (42.0588, -35.1471) radius 1.5
  circle A514 centre (48.9706, -35.1471) radius 1.5
  circle A515 centre (55.8824, -35.1471) radius 1.5
  circle A516 centre (62.7941, -35.1471) radius 1.5
  circle A517 centre (69.7059, -35.1471) radius 1.5
  circle A518 centre (76.6176, -35.1471) radius 1.5
  circle A519 centre (83.5294, -35.1471) radius 1.5
  circle A520 centre (90.4412, -35.1471) radius 1.5
  circle A521 centre (97.3529, -35.1471) radius 1.5
  circle A522 centre (104.2647, -35.1471) radius 1.5
  circle A523 centre (111.1765, -35.1471) radius 1.5
  circle A524 centre (118.0882, -35.1471) radius 1.5
  circle A525 centre (125, -35.1471) radius 1.5
  circle A526 centre (131.9118, -35.1471) radius 1.5
  circle A527 centre (138.8235, -35.1471) radius 1.5
  circle A528 centre (145.7353, -35.1471) radius 1.5
  circle A529 centre (152.6471, -35.1471) radius 1.5
  circle A530 centre (159.5588, -35.1471) radius 1.5
  circle A531 centre (166.4706, -35.1471) radius 1.5
  circle A532 centre (173.3824, -35.1471) radius 1.5
  circle A533 centre (180.2941, -35.1471) radius 1.5
  circle A534 centre (187.2059, -35.1471) radius 1.5
  circle A535 centre (194.1176, -35.1471) radius 1.5
  circle A536 centre (201.0294, -35.1471) radius 1.5
  circle A537 centre (207.9412, -35.1471) radius 1.5
  circle A538 centre (214.8529, -35.1471) radius 1.5
  circle A539 centre (221.7647, -35.1471) radius 1.5
  circle A540 centre (228.6765, -35.1471) radius 1.5
  circle A541 centre (235.5882, -35.1471) radius 1.5
  circle A542 centre (242.5, -35.1471) radius 1.5
  circle A543 centre (14.4118, -42.0588) radius 1.5
  circle A544 centre (21.3235, -42.0588) radius 1.5
  circle A545 centre (28.2353, -42.0588) radius 1.5
  circle A546 centre (35.1471, -42.0588) radius 1.5
  circle A547 centre (42.0588, -42.0588) radius 1.5
  circle A548 centre (48.9706, -42.0588) radius 1.5
  circle A549 centre (55.8824, -42.0588) radius 1.5
  circle A550 centre (62.7941, -42.0588) radius 1.5
  circle A551 centre (69.7059, -42.0588) radius 1.5
  circle A552 centre (76.6176, -42.0588) radius 1.5
  circle A553 centre (83.5294, -42.0588) radius 1.5
  circle A554 centre (90.4412, -42.0588) radius 1.5
  circle A555 centre (97.3529, -42.0588) radius 1.5
  circle A556 centre (104.2647, -42.0588) radius 1.5
  circle A557 centre (111.1765, -42.0588) radius 1.5
  circle A558 centre (118.0882, -42.0588) radius 1.5
  circle A559 centre (125, -42.0588) radius 1.5
  circle A560 centre (131.9118, -42.0588) radius 1.5
  circle A561 centre (138.8235, -42.0588) radius 1.5
  circle A562 centre (145.7353, -42.0588) radius 1.5
  circle A563 centre (152.6471, -42.0588) radius 1.5
  circle A564 centre (159.5588, -42.0588) radius 1.5
  circle A565 centre (166.4706, -42.0588) radius 1.5
  circle A566 centre (173.3824, -42.0588) radius 1.5
  circle A567 centre (180.2941, -42.0588) radius 1.5
  circle A568 centre (187.2059, -42.0588) radius 1.5
  circle A569 centre (194.1176, -42.0588) radius 1.5
  circle A570 centre (201.0294, -42.0588) radius 1.5
  circle A571 centre (207.9412, -42.0588) radius 1.5
  circle A572 centre (214.8529, -42.0588) radius 1.5
  circle A573 centre (221.7647, -42.0588) radius 1.5
  circle A574 centre (228.6765, -42.0588) radius 1.5
  circle A575 centre (235.5882, -42.0588) radius 1.5
  circle A576 centre (242.5, -42.0588) radius 1.5
  circle A577 centre (14.4118, -48.9706) radius 1.5
  circle A578 centre (21.3235, -48.9706) radius 1.5
  circle A579 centre (28.2353, -48.9706) radius 1.5
  circle A580 centre (35.1471, -48.9706) radius 1.5
  circle A581 centre (42.0588, -48.9706) radius 1.5
  circle A582 centre (48.9706, -48.9706) radius 1.5
  circle A583 centre (55.8824, -48.9706) radius 1.5
  circle A584 centre (62.7941, -48.9706) radius 1.5
  circle A585 centre (69.7059, -48.9706) radius 1.5
  circle A586 centre (76.6176, -48.9706) radius 1.5
  circle A587 centre (83.5294, -48.9706) radius 1.5
  circle A588 centre (90.4412, -48.9706) radius 1.5
  circle A589 centre (97.3529, -48.9706) radius 1.5
  circle A590 centre (104.2647, -48.9706) radius 1.5
  circle A591 centre (111.1765, -48.9706) radius 1.5
  circle A592 centre (118.0882, -48.9706) radius 1.5
  circle A593 centre (125, -48.9706) radius 1.5
  circle A594 centre (131.9118, -48.9706) radius 1.5
  circle A595 centre (138.8235, -48.9706) radius 1.5
  circle A596 centre (145.7353, -48.9706) radius 1.5
  circle A597 centre (152.6471, -48.9706) radius 1.5
  circle A598 centre (159.5588, -48.9706) radius 1.5
  circle A599 centre (166.4706, -48.9706) radius 1.5
  circle A600 centre (173.3824, -48.9706) radius 1.5
  circle A601 centre (180.2941, -48.9706) radius 1.5
  circle A602 centre (187.2059, -48.9706) radius 1.5
  circle A603 centre (194.1176, -48.9706) radius 1.5
  circle A604 centre (201.0294, -48.9706) radius 1.5
  circle A605 centre (207.9412, -48.9706) radius 1.5
  circle A606 centre (214.8529, -48.9706) radius 1.5
  circle A607 centre (221.7647, -48.9706) radius 1.5
  circle A608 centre (228.6765, -48.9706) radius 1.5
  circle A609 centre (235.5882, -48.9706) radius 1.5
  circle A610 centre (242.5, -48.9706) radius 1.5
  circle A611 centre (14.4118, -55.8824) radius 1.5
  circle A612 centre (21.3235, -55.8824) radius 1.5
  circle A613 centre (28.2353, -55.8824) radius 1.5
  circle A614 centre (35.1471, -55.8824) radius 1.5
  circle A615 centre (42.0588, -55.8824) radius 1.5
  circle A616 centre (48.9706, -55.8824) radius 1.5
  circle A617 centre (55.8824, -55.8824) radius 1.5
  circle A618 centre (62.7941, -55.8824) radius 1.5
  circle A619 centre (69.7059, -55.8824) radius 1.5
  circle A620 centre (76.6176, -55.8824) radius 1.5
  circle A621 centre (83.5294, -55.8824) radius 1.5
  circle A622 centre (90.4412, -55.8824) radius 1.5
  circle A623 centre (97.3529, -55.8824) radius 1.5
  circle A624 centre (104.2647, -55.8824) radius 1.5
  circle A625 centre (111.1765, -55.8824) radius 1.5
  circle A626 centre (118.0882, -55.8824) radius 1.5
  circle A627 centre (125, -55.8824) radius 1.5
  circle A628 centre (131.9118, -55.8824) radius 1.5
  circle A629 centre (138.8235, -55.8824) radius 1.5
  circle A630 centre (145.7353, -55.8824) radius 1.5
  circle A631 centre (152.6471, -55.8824) radius 1.5
  circle A632 centre (159.5588, -55.8824) radius 1.5
  circle A633 centre (166.4706, -55.8824) radius 1.5
  circle A634 centre (173.3824, -55.8824) radius 1.5
  circle A635 centre (180.2941, -55.8824) radius 1.5
  circle A636 centre (187.2059, -55.8824) radius 1.5
  circle A637 centre (194.1176, -55.8824) radius 1.5
  circle A638 centre (201.0294, -55.8824) radius 1.5
  circle A639 centre (207.9412, -55.8824) radius 1.5
  circle A640 centre (214.8529, -55.8824) radius 1.5
  circle A641 centre (221.7647, -55.8824) radius 1.5
  circle A642 centre (228.6765, -55.8824) radius 1.5
  circle A643 centre (235.5882, -55.8824) radius 1.5
  circle A644 centre (242.5, -55.8824) radius 1.5
  circle A645 centre (14.4118, -62.7941) radius 1.5
  circle A646 centre (21.3235, -62.7941) radius 1.5
  circle A647 centre (28.2353, -62.7941) radius 1.5
  circle A648 centre (35.1471, -62.7941) radius 1.5
  circle A649 centre (42.0588, -62.7941) radius 1.5
  circle A650 centre (48.9706, -62.7941) radius 1.5
  circle A651 centre (55.8824, -62.7941) radius 1.5
  circle A652 centre (62.7941, -62.7941) radius 1.5
  circle A653 centre (69.7059, -62.7941) radius 1.5
  circle A654 centre (76.6176, -62.7941) radius 1.5
  circle A655 centre (83.5294, -62.7941) radius 1.5
  circle A656 centre (90.4412, -62.7941) radius 1.5
  circle A657 centre (97.3529, -62.7941) radius 1.5
  circle A658 centre (104.2647, -62.7941) radius 1.5
  circle A659 centre (111.1765, -62.7941) radius 1.5
  circle A660 centre (118.0882, -62.7941) radius 1.5
  circle A661 centre (125, -62.7941) radius 1.5
  circle A662 centre (131.9118, -62.7941) radius 1.5
  circle A663 centre (138.8235, -62.7941) radius 1.5
  circle A664 centre (145.7353, -62.7941) radius 1.5
  circle A665 centre (152.6471, -62.7941) radius 1.5
  circle A666 centre (159.5588, -62.7941) radius 1.5
  circle A667 centre (166.4706, -62.7941) radius 1.5
  circle A668 centre (173.3824, -62.7941) radius 1.5
  circle A669 centre (180.2941, -62.7941) radius 1.5
  circle A670 centre (187.2059, -62.7941) radius 1.5
  circle A671 centre (194.1176, -62.7941) radius 1.5
  circle A672 centre (201.0294, -62.7941) radius 1.5
  circle A673 centre (207.9412, -62.7941) radius 1.5
  circle A674 centre (214.8529, -62.7941) radius 1.5
  circle A675 centre (221.7647, -62.7941) radius 1.5
  circle A676 centre (228.6765, -62.7941) radius 1.5
  circle A677 centre (235.5882, -62.7941) radius 1.5
  circle A678 centre (242.5, -62.7941) radius 1.5
  circle A679 centre (14.4118, -69.7059) radius 1.5
  circle A680 centre (21.3235, -69.7059) radius 1.5
  circle A681 centre (28.2353, -69.7059) radius 1.5
  circle A682 centre (35.1471, -69.7059) radius 1.5
  circle A683 centre (42.0588, -69.7059) radius 1.5
  circle A684 centre (48.9706, -69.7059) radius 1.5
  circle A685 centre (55.8824, -69.7059) radius 1.5
  circle A686 centre (62.7941, -69.7059) radius 1.5
  circle A687 centre (69.7059, -69.7059) radius 1.5
  circle A688 centre (76.6176, -69.7059) radius 1.5
  circle A689 centre (83.5294, -69.7059) radius 1.5
  circle A690 centre (90.4412, -69.7059) radius 1.5
  circle A691 centre (97.3529, -69.7059) radius 1.5
  circle A692 centre (104.2647, -69.7059) radius 1.5
  circle A693 centre (111.1765, -69.7059) radius 1.5
  circle A694 centre (118.0882, -69.7059) radius 1.5
  circle A695 centre (125, -69.7059) radius 1.5
  circle A696 centre (131.9118, -69.7059) radius 1.5
  circle A697 centre (138.8235, -69.7059) radius 1.5
  circle A698 centre (145.7353, -69.7059) radius 1.5
  circle A699 centre (152.6471, -69.7059) radius 1.5
  circle A700 centre (159.5588, -69.7059) radius 1.5
  circle A701 centre (166.4706, -69.7059) radius 1.5
  circle A702 centre (173.3824, -69.7059) radius 1.5
  circle A703 centre (180.2941, -69.7059) radius 1.5
  circle A704 centre (187.2059, -69.7059) radius 1.5
  circle A705 centre (194.1176, -69.7059) radius 1.5
  circle A706 centre (201.0294, -69.7059) radius 1.5
  circle A707 centre (207.9412, -69.7059) radius 1.5
  circle A708 centre (214.8529, -69.7059) radius 1.5
  circle A709 centre (221.7647, -69.7059) radius 1.5
  circle A710 centre (228.6765, -69.7059) radius 1.5
  circle A711 centre (235.5882, -69.7059) radius 1.5
  circle A712 centre (242.5, -69.7059) radius 1.5
  circle A713 centre (14.4118, -76.6176) radius 1.5
  circle A714 centre (21.3235, -76.6176) radius 1.5
  circle A715 centre (28.2353, -76.6176) radius 1.5
  circle A716 centre (35.1471, -76.6176) radius 1.5
  circle A717 centre (42.0588, -76.6176) radius 1.5
  circle A718 centre (48.9706, -76.6176) radius 1.5
  circle A719 centre (55.8824, -76.6176) radius 1.5
  circle A720 centre (62.7941, -76.6176) radius 1.5
  circle A721 centre (69.7059, -76.6176) radius 1.5
  circle A722 centre (76.6176, -76.6176) radius 1.5
  circle A723 centre (83.5294, -76.6176) radius 1.5
  circle A724 centre (90.4412, -76.6176) radius 1.5
  circle A725 centre (97.3529, -76.6176) radius 1.5
  circle A726 centre (104.2647, -76.6176) radius 1.5
  circle A727 centre (111.1765, -76.6176) radius 1.5
  circle A728 centre (118.0882, -76.6176) radius 1.5
  circle A729 centre (125, -76.6176) radius 1.5
  circle A730 centre (131.9118, -76.6176) radius 1.5
  circle A731 centre (138.8235, -76.6176) radius 1.5
  circle A732 centre (145.7353, -76.6176) radius 1.5
  circle A733 centre (152.6471, -76.6176) radius 1.5
  circle A734 centre (159.5588, -76.6176) radius 1.5
  circle A735 centre (166.4706, -76.6176) radius 1.5
  circle A736 centre (173.3824, -76.6176) radius 1.5
  circle A737 centre (180.2941, -76.6176) radius 1.5
  circle A738 centre (187.2059, -76.6176) radius 1.5
  circle A739 centre (194.1176, -76.6176) radius 1.5
  circle A740 centre (201.0294, -76.6176) radius 1.5
  circle A741 centre (207.9412, -76.6176) radius 1.5
  circle A742 centre (214.8529, -76.6176) radius 1.5
  circle A743 centre (221.7647, -76.6176) radius 1.5
  circle A744 centre (228.6765, -76.6176) radius 1.5
  circle A745 centre (235.5882, -76.6176) radius 1.5
  circle A746 centre (242.5, -76.6176) radius 1.5